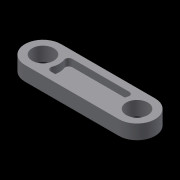
# Autodesk Inventor part: SpineTopMiddleConnector
Saved by Autodesk Inventor 2015 (Build 190159000, 159)
## iProperties
Created: 2015-01-13
Part Number: SpineTopMiddleConnector
Material: Generic
Document SubType Name: Modeling
Designer: Val
Density: 1 g/cm^3
Appearance: Default
Mass: 0.862182 g
Surface Area: 11.3633 cm^2
Volume: 0.862182 cm^3
Author: Val
Autodesk Inventor part; units mm, degrees
ref_plane "YZ Plane" through (0, 0, 0) normal (1, 0, 0) x (0, 1, 0)
ref_plane "XZ Plane" through (0, 0, 0) normal (0, 1, 0) x (-1, 0, 0)
ref_plane "XY Plane" through (0, 0, 0) normal (0, 0, 1) x (1, 0, 0)
sketch "Base" plane through (0, 0, 0) normal (0, 0, 1) x (1, 0, 0)
  circle A0 centre (0, 0) radius 5
  circle A1 centre (0, 0) radius 3
  line L0 (0, 0) -> (-26, 0) construction
  circle A2 centre (-26, 0) radius 5
  circle A3 centre (-26, 0) radius 3
  line L1 (-26, 5) -> (0, 5)
  line L2 (-26, -5) -> (0, -5)
  line L3 (-26, 3) -> (0, 3)
  line L4 (-26, -3) -> (0, -3)
  dimension "d0" = 10
  dimension "d1" = 6
  dimension "d2" = 26
  dimension "d7" = 10
  constraints: 10 end point, 8 point on circle, 8 tangent, 4 centre point, 4 coincident, 1 equal radius, 1 horizontal
  measures "d0" diameter of A0
  measures "d1" diameter of A1
  measures "d2" distance of L0.start L0.end
  measures "d7" diameter of A2
extrude "BaseFeature" add sketch "Base" along normal blind 4 contours A0 L4 A1 L3 | A0 L3 A2 L1 | L2 A2 L4 A0 | L3 A1 L4 A0 | A0 L4 A2 L3 | A2 L3 A3 L4 | A2 L4 A3 L3
sketch "Inset" plane through (0, 0, 4) normal (0, 0, 1) x (1, 0, 0)
  circle A0 centre (-26, 0) radius 3 projected
  circle A1 centre (0, 0) radius 3 projected
  circle A2 centre (-26, 0) radius 3 projected
  line L0 (-26, 3) -> (0, 3)
  circle A3 centre (0, 0) radius 3 projected
  line L1 (-26, -3) -> (0, -3)
  constraints: 8 point on circle, 4 end point, 4 tangent
extrude "InsetFeature" cut sketch "Inset" against normal blind 2 contours A0 L0 A1 L1
sketch "HoleBorders" plane through (0, 0, 0) normal (0, 0, -1) x (-1, 0, 0)
  circle A0 centre (0, 0) radius 3 projected
  circle A1 centre (26, 0) radius 3 projected
  circle A2 centre (0, 0) radius 4.5
  circle A3 centre (26, 0) radius 4.5
  dimension "d13" = 9
  dimension "d14" = 9
  constraints: 2 centre point, 2 coincident
  measures "d13" diameter of A2
  measures "d14" diameter of A3
extrude "HoleBordersFeature" add sketch "HoleBorders" against normal up to surface (4 mm away)
fillet "HoleBorderFilletsFeature" radius 1 4 edges at (-3.3541, -3, 3) (-3.3541, 3, 3) (-22.6459, -3, 3) (-22.6459, 3, 3)
